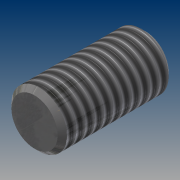
# Autodesk Inventor part: M6_12mm
Saved by Autodesk Inventor 2015 SP1 (Build 190203100, 203)
## iProperties
Created: 2015-03-27
Part Number: M6_12mm
Material: Steel, Carbon
Document SubType Name: Modeling
Designer: nfitch
Density: 7.85 g/cm^3
Appearance: Semi-Polished
Mass: 5.07153 g
Surface Area: 6.60754 cm^2
Volume: 0.646055 cm^3
Author: nfitch
Autodesk Inventor part; units mm, degrees
ref_plane "YZ Plane" through (0, 0, 0) normal (1, 0, 0) x (0, 1, 0)
ref_plane "XZ Plane" through (0, 0, 0) normal (0, 1, 0) x (-1, 0, 0)
ref_plane "XY Plane" through (0, 0, 0) normal (0, 0, 1) x (1, 0, 0)
sketch "Sketch1" plane through (0, 0, 0) normal (0, 1, 0) x (-1, 0, 0)
  circle A0 centre (0, 0) radius 3
  dimension "d0" = 6
  constraints: 1 centre point, 1 coincident
  measures "d0" diameter of A0
extrude "Extrusion1" add sketch "Sketch1" along normal blind 12
thread "Thread1" size "M6x1" class "6g" standard "ANSI Metric M Profile" full length
chamfer "Chamfer1" distance 0.5 angle 45 2 edges at (3, 0, 0) (3, 12, 0)
body "Solid1"
